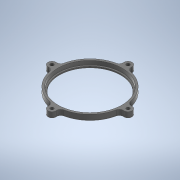
# Autodesk Inventor part: BearingClamp
Saved by Autodesk Inventor 2020 (Build 240168000, 168)
## iProperties
Created: 2019-05-28
Part Number: BearingClamp
Material: ABS Plastic
Document SubType Name: Modeling
Designer: Connor
Density: 1.06 g/cm^3
Appearance: Smooth - Black
Author: Connor
Autodesk Inventor part; units mm, degrees
ref_plane "YZ Plane" through (0, 0, 0) normal (1, 0, 0) x (0, 1, 0)
ref_plane "XZ Plane" through (0, 0, 0) normal (0, 1, 0) x (-1, 0, 0)
ref_plane "XY Plane" through (0, 0, 0) normal (0, 0, 1) x (1, 0, 0)
sketch "Sketch1" plane through (0, 0, 0) normal (0, 0, 1) x (1, 0, 0)
  line L0 (0, 0) -> (50.8, 0) construction
  line L1 (50.8, 0) -> (50.8, -6.35) construction
  line L2 (50.8, -6.35) -> (0, -6.35) construction
  line L3 (0, -6.35) -> (0, 0) construction
  line L4 (50.8, -6.35) -> (48.26, -6.35)
  line L5 (48.26, -6.35) -> (48.26, -9.525)
  line L6 (48.26, -9.525) -> (50.8, -9.525)
  line L7 (50.8, -9.525) -> (50.8, -6.35)
  line L8 (50.8, 0) -> (53.975, 0)
  line L9 (53.975, 0) -> (53.975, -9.525)
  line L10 (53.975, -9.525) -> (50.8, -9.525)
  line L11 (50.8, -9.525) -> (50.8, 0)
  dimension "d0" = 50.8
  dimension "d2" = 6.35
  dimension "d3" = 2.54
  dimension "d4" = 3.175
  dimension "d5" = 9.525
  constraints: 24 end point, 4 parallel, 4 perpendicular, 3 horizontal, 1 collinear, 1 vertical
  measures "d0" distance of L0.start L0.end
  measures "d2" distance of L2.end L0.start
  measures "d3" distance between parallel lines of L7 L5
  measures "d4" distance of L0.end L8.end
  measures "d5" distance of L8.end L9.end
revolve "Revolution1" add sketch "Sketch1" angle 360 about axis through (0, -6.35, 0) along (0, 1, 0)
sketch "Sketch2" plane through (0, 0, 0) normal (0, 1, 0) x (-1, 0, 0)
  circle A0 centre (0, 0) radius 53.975 projected
  circle A1 centre (0, -60.325) radius 6.35
  circle A2 centre (0, 0) radius 53.975 projected
  circle A3 centre (12.6294, -58.9882) radius 6.35 construction
  circle A4 centre (-12.6294, -58.9882) radius 6.35 construction
  circle A5 centre (0, -60.325) radius 2.5797
  arc A6 (11.3, -52.7789) -> (6.3147, -59.6566) centre (12.6294, -58.9882) ccw
  arc A7 (-6.3147, -59.6566) -> (-11.3, -52.7789) centre (-12.6294, -58.9882) ccw
  point P0 (11.3, -52.7789)
  point P1 (-11.3, -52.7789)
  dimension "d7" = 5.1594
  dimension "d14" = 12.7
  constraints: 12 point on circle, 6 centre point, 5 tangent, 3 coincident, 2 equal radius, 1 vertical alignment
  measures "d7" diameter of A5
  measures "d14" diameter of A1
extrude "Extrusion1" add sketch "Sketch2" against normal up to surface (9.525 mm away) contours A0 A1 A7 | A6 A1 A0 | A1
pattern_circular "Circular Pattern1" count 4 over 360 about axis through (0, -10, 0) along (0, 1, 0) of "Extrusion1"
fillet "Fillet1" radius 1.5875 5 edges at (-48.26, -9.525, 0) (-38.1661, -9.525, -38.1661) (-38.1661, -9.525, 38.1661) (38.1661, -9.525, 38.1661) (38.1661, -9.525, -38.1661)
body "Solid1"
